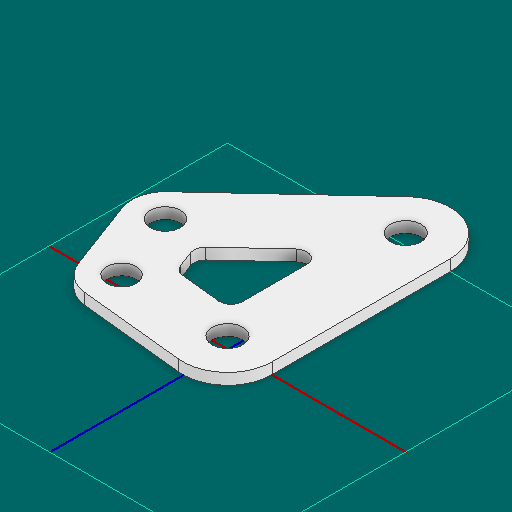
# Autodesk Inventor part: mount
Saved by Autodesk Inventor 2025 (Build 290162000, 162)
## iProperties
Created: 2024-08-21
Part Number: mount
Material: Acetal Resin, White
Document SubType Name: Modeling
Designer: averey
Density: 1.425 g/cm^3
Appearance: Smooth - White
Author: averey
Autodesk Inventor part; units mm, degrees
ref_plane "YZ Plane" through (0, 0, 0) normal (1, 0, 0) x (0, 1, 0)
ref_plane "XZ Plane" through (0, 0, 0) normal (0, 1, 0) x (-1, 0, 0)
ref_plane "XY Plane" through (0, 0, 0) normal (0, 0, 1) x (1, 0, 0)
sketch "main" plane through (0, 0, 0) normal (0, 0, 1) x (1, 0, 0)
  circle A0 centre (15.4343, 10.6591) radius 2.1844
  circle A1 centre (5.3986, -8.2031) radius 2.15
  circle A2 centre (-9.9657, 10.6591) radius 2.1844
  circle A3 centre (15.4343, -4.4222) radius 2.0955
  arc A4 (17.1111, -8.9158) -> (20.205, -4.9163) centre (15.4343, -4.4222) ccw
  arc A5 (21.7505, 10.0049) -> (15.4343, 17.0091) centre (15.4343, 10.6591) ccw
  arc A6 (-9.9657, 17.0091) -> (-14.6169, 6.336) centre (-9.9657, 10.6591) ccw
  arc A7 (1.9103, -11.4454) -> (7.0637, -12.6651) centre (5.3986, -8.2031) ccw
  line L0 (21.7505, 10.0049) -> (20.205, -4.9163)
  line L1 (15.4343, 17.0091) -> (-9.9657, 17.0091)
  line L2 (-14.6169, 6.336) -> (1.9103, -11.4454)
  line L3 (17.1111, -8.9158) -> (7.0637, -12.6651)
  line L4 (7.7131, -2.2562) -> (10.1103, -1.3616)
  line L5 (11.1343, -0.0379) -> (11.7321, 5.733)
  line L6 (10.153, 7.4841) -> (0.9628, 7.4841)
  line L7 (-0.2, 4.8158) -> (5.9953, -1.8496)
  arc A8 (10.1103, -1.3616) -> (11.1343, -0.0379) centre (9.5553, 0.1257) ccw
  arc A9 (5.9953, -1.8496) -> (7.7131, -2.2562) centre (7.1581, -0.7688) ccw
  arc A10 (0.9628, 7.4841) -> (-0.2, 4.8158) centre (0.9628, 5.8966) ccw
  arc A11 (11.7321, 5.733) -> (10.153, 7.4841) centre (10.153, 5.8966) ccw
  point P0 (7.047, 1.8005)
  dimension "d0" = 4.191
  dimension "d1" = 12.7
  dimension "d2" = 12.7
  dimension "d3" = 9.525
  dimension "d4" = 9.525
  dimension "d5" = 1.5875
  measures "d0" diameter of A3
  measures "d1" diameter of A6
  measures "d2" diameter of A5
  measures "d3" diameter of A7
  measures "d4" distance between parallel lines of L3 L4
  measures "d5" radius of A8
sketch "Sketch1" plane through (0, 0, 0) normal (0, 1, 0) x (-1, 0, 0)
  circle A0 centre (0, 0) radius 2.1844
  circle A1 centre (18.8698, -10.0212) radius 2.15
  circle A2 centre (0.0195, -25.4) radius 2.1844
  circle A3 centre (15.0812, 0.0116) radius 2.0955
  arc A4 (19.5736, 1.6918) -> (15.5717, 4.7827) centre (15.0812, 0.0116) ccw
  arc A5 (0.6494, 6.3167) -> (-6.35, -0.0049) centre (0, 0) ccw
  arc A6 (-6.3305, -25.4049) -> (4.3461, -30.0478) centre (0.0195, -25.4) ccw
  arc A7 (22.1148, -13.507) -> (23.3305, -8.3527) centre (18.8698, -10.0212) ccw
  line L0 (0.6494, 6.3167) -> (15.5717, 4.7827)
  line L1 (-6.35, -0.0049) -> (-6.3305, -25.4049)
  line L2 (4.3461, -30.0478) -> (22.1148, -13.507)
  line L3 (19.5736, 1.6918) -> (23.3305, -8.3527)
  line L4 (12.9211, -7.7113) -> (12.0248, -5.3147)
  line L5 (10.7002, -4.2917) -> (4.9289, -3.6984)
  line L6 (3.179, -5.2788) -> (3.1861, -14.469)
  line L7 (5.8553, -15.6297) -> (12.5159, -9.4294)
  arc A8 (12.0248, -5.3147) -> (10.7002, -4.2917) centre (10.5379, -5.8709) ccw
  arc A9 (12.5159, -9.4294) -> (12.9211, -7.7113) centre (11.4342, -8.2674) ccw
  arc A10 (3.1861, -14.469) -> (5.8553, -15.6297) centre (4.7736, -14.4678) ccw
  arc A11 (4.9289, -3.6984) -> (3.179, -5.2788) centre (4.7665, -5.2776) ccw
  point P0 (0, 0)
  constraints: 1 other
extrude "Extrusion1" add sketch "Sketch1" along normal blind 1.5875
body "Solid1"
